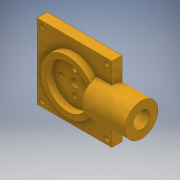
# Autodesk Inventor part: NewGimbalPart4
Saved by Autodesk Inventor 2017 SP1 (Build 210196100, 196)
## iProperties
Created: 2019-10-30
Part Number: NewGimbalPart4
Material: Brass, Soft Yellow, Welded
Document SubType Name: Modeling
Designer: h34sh00ters4m
Density: 8.5 g/cm^3
Appearance: Weld - Brass
Author: h34sh00ters4m
Autodesk Inventor part; units mm, degrees
ref_plane "YZ Plane" through (0, 0, 0) normal (1, 0, 0) x (0, 1, 0)
ref_plane "XZ Plane" through (0, 0, 0) normal (0, 1, 0) x (-1, 0, 0)
ref_plane "XY Plane" through (0, 0, 0) normal (0, 0, 1) x (1, 0, 0)
sketch "Sketch1" plane through (0, 0, 0) normal (0, 1, 0) x (-1, 0, 0)
  circle A0 centre (0, 0) radius 14.8
  circle A1 centre (0, 0) radius 18.6876
  dimension "d0" = 29.6
  constraints: 2 centre point, 2 coincident
  measures "d0" diameter of A0
extrude "Extrusion1" add sketch "Sketch1" along normal blind 5
sketch "Sketch2" plane through (0, 5, 0) normal (0, 1, 0) x (1, 0, 0)
  line L0 (0, 0) -> (0, 26)
  line L1 (0, 26) -> (-26, 26)
  line L2 (-26, 26) -> (-26, -26)
  line L3 (-26, -26) -> (26, -26)
  line L4 (26, -26) -> (26, 26)
  line L5 (26, 26) -> (-26, 26)
  line L6 (-26, 26) -> (-26, -26)
  dimension "d3" = 26
  dimension "d4" = 26
  dimension "d5" = 52
  dimension "d6" = 52
  constraints: 14 end point, 3 perpendicular, 2 parallel, 1 horizontal, 1 vertical
  measures "d3" distance of L0.start L0.end
  measures "d4" distance of L0.end L1.end
  measures "d5" distance of L1.end L2.end
  measures "d6" distance of L5.end L4.end
extrude "Extrusion2" add sketch "Sketch2" along normal blind 7
sketch "Sketch3" plane through (0, 5, 0) normal (0, -1, 0) x (1, 0, 0)
  circle A0 centre (9.5, 0) radius 1.8
  circle A1 centre (-9.5, 0) radius 1.8
  circle A2 centre (0, -8) radius 1.8
  circle A3 centre (0, 8) radius 1.8
  circle A4 centre (0, 0) radius 3
  dimension "d11" = 3.6
  dimension "d12" = 3.6
  dimension "d13" = 3.6
  dimension "d14" = 3.6
  dimension "d15" = 6
  constraints: 5 centre point, 1 coincident
  measures "d11" diameter of A0
  measures "d12" diameter of A1
  measures "d13" diameter of A2
  measures "d14" diameter of A3
  measures "d15" diameter of A4
extrude "Extrusion3" cut sketch "Sketch3" against normal blind 15
sketch "Sketch4" plane through (26, 5, 26) normal (1, 0, 0) x (0, 0, -1)
  line L0 (52, 0) -> (0, 0) projected
  line L1 (26, 0) -> (26, 1)
  circle A0 centre (26, 1) radius 5.8
  circle A1 centre (26, 1) radius 11.4632
  point P0 (26, -5)
  dimension "d18" = 1
  dimension "d19" = 11.6
  constraints: 2 centre point, 2 coincident, 2 end point, 1 midpoint, 1 vertical
  measures "d18" distance of L1.start L1.end
  measures "d19" diameter of A0
extrude "Extrusion4" add sketch "Sketch4" along normal blind 19.5 and the other way blind 10.5 contours A1 L0 A0 | L0 A0 A1
sketch "Sketch5" plane through (45.5, 6, 0) normal (1, 0, 0) x (0, 0, -1)
  circle A0 centre (0, 0) radius 5.8 projected
  circle A1 centre (0, 0) radius 5.8
  point P0 (0, -6)
  constraints: 1 centre point, 1 coincident
extrude "Extrusion5" cut sketch "Sketch5" against normal blind 32
sketch "Sketch6" plane through (0, 12, 0) normal (0, 1, 0) x (1, 0, 0)
  line L0 (0, 0) -> (0, 22.5)
  line L1 (0, 22.5) -> (-22.5, 22.5)
  line L2 (-22.5, 22.5) -> (-22.5, -22.5)
  line L3 (-22.5, -22.5) -> (22.5, -22.5)
  line L4 (22.5, -22.5) -> (22.5, 22.5)
  circle A0 centre (-22.5, 22.5) radius 1.8
  circle A1 centre (22.5, 22.5) radius 1.8
  circle A2 centre (-22.5, -22.5) radius 1.8
  circle A3 centre (22.5, -22.5) radius 1.8
  dimension "d26" = 22.5
  dimension "d27" = 22.5
  dimension "d28" = 45
  dimension "d29" = 45
  dimension "d30" = 3.6
  dimension "d31" = 3.6
  dimension "d32" = 3.6
  dimension "d33" = 3.6
  constraints: 10 end point, 4 centre point, 4 coincident, 4 perpendicular, 1 point on line, 1 vertical
  measures "d26" distance of L0.start L0.end
  measures "d27" distance of L0.end L1.end
  measures "d28" distance of L1.end L2.end
  measures "d29" distance of L2.end L3.end
  measures "d30" diameter of A0
  measures "d31" diameter of A1
  measures "d32" diameter of A2
  measures "d33" diameter of A3
extrude "Extrusion6" cut sketch "Sketch6" against normal blind 32
body "Solid1"
